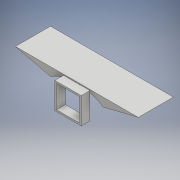
# Autodesk Inventor part: RescueKitThrow_slope
Saved by Autodesk Inventor 2018.3 (Build 223284000, 284)
## iProperties
Created: 2019-02-15
Part Number: RescueKitThrow_slope
Material: 一般
Document SubType Name: Modeling
Designer: TOMOKI
Density: 1 g/cm^3
Appearance: 既定
Author: TOMOKI
Autodesk Inventor part; units mm, degrees
ref_plane "YZ Plane" through (0, 0, 0) normal (1, 0, 0) x (0, 1, 0)
ref_plane "XZ Plane" through (0, 0, 0) normal (0, 1, 0) x (-1, 0, 0)
ref_plane "XY Plane" through (0, 0, 0) normal (0, 0, 1) x (1, 0, 0)
sketch "スケッチ1" plane through (0, 0, 0) normal (0, 1, 0) x (-1, 0, 0)
  line L0 (55, 0) -> (85, 0)
  line L1 (57, -2) -> (83, -2)
  line L2 (83, -2) -> (83, -28)
  line L3 (83, -28) -> (57, -28)
  line L4 (57, -28) -> (57, -2)
  line L5 (85, -30) -> (55, -30)
  line L6 (55, -30) -> (55, 0)
  line L7 (85, 0) -> (85, -30)
  point P0 (0, 0)
  dimension "d15" = 30
  constraints: 16 end point
  measures "d15" distance of L0.end L0.start
extrude "押し出し1" add sketch "スケッチ1" along normal blind 10
sketch "スケッチ3" plane through (0, 10, 0) normal (0, 1, 0) x (1, 0, 0)
  line L0 (0, 0) -> (-140, 0)
  line L1 (0, 0) -> (0, -8.775)
  line L2 (-140, 8.775) -> (-140, 38.775)
  line L3 (-140, 38.775) -> (0, 38.775)
  line L4 (0, 38.775) -> (0, 0)
  line L5 (-140, 0) -> (-140, 38.775)
  line L6 (0, 0) -> (0, 8.775)
  line L7 (0, 8.775) -> (-40.1965, 8.775)
  line L8 (0, 8.775) -> (-40.1965, 8.775)
  line L9 (-99.8035, 8.775) -> (-140, 8.775)
  line L10 (-99.8035, 8.775) -> (-140, 8.775)
  arc A0 (-99.8035, 8.775) -> (-40.1965, 8.775) centre (-70, 55) ccw
  point P0 (-140, -38.775)
  point P1 (-40.1965, -8.775)
  constraints: 22 end point, 3 symmetric about line, 2 point on circle, 1 centre point, 1 point on line
extrude "押し出し2" add sketch "スケッチ3" along normal blind 40 contours L0 A0 L7 L4 | L0 L5 L9 A0
sketch "スケッチ4" plane through (0, 10, 0) normal (0, 0, 1) x (1, 0, 0)
  line L0 (0, 40) -> (-140, 40)
  line L1 (-140, 40) -> (-140, 0)
  line L2 (-140, 0) -> (0, 0)
  line L3 (0, 0) -> (0, 40)
  point P0 (0, -10)
  constraints: 8 end point, 2 parallel, 1 horizontal, 1 perpendicular
extrude "押し出し3" add sketch "スケッチ4" along normal blind 1
sketch "スケッチ5" plane through (0, 50, 0) normal (0, 1, 0) x (1, 0, 0)
  line L0 (0, -1) -> (0, 8.775) projected
  line L1 (-140, 8.775) -> (-140, -1) projected
  line L2 (-99.8035, 8.775) -> (-140, 8.775) projected
  line L3 (-140, 8.775) -> (-140, -1) projected
  line L4 (0, -1) -> (-140, -1) projected
  line L5 (0, 8.775) -> (0, -1) projected
  line L6 (0, 8.775) -> (-40.1965, 8.775) projected
  arc A0 (-99.8035, 8.775) -> (-40.1965, 8.775) centre (-70, 55) ccw projected
  line L7 (-140, -1) -> (0, -1) projected
  line L8 (-40.1965, 8.775) -> (0, -1)
  arc A1 (-99.8035, 8.775) -> (-40.1965, 8.775) centre (-70, 55) ccw projected
  line L9 (-99.8035, 8.775) -> (-140, -1)
  constraints: 4 end point
extrude "押し出し4" cut sketch "スケッチ5" against normal blind 40 contours L8 L6 L0 | L1 L2 L9
sketch "スケッチ6" plane through (0, 10, 0) normal (0, 1, 0) x (1, 0, 0)
  line L0 (0, -8.775) -> (-40.1965, -8.775) projected
  line L1 (-57, 28) -> (-57, 2) projected
  line L2 (-40.1965, -8.775) -> (-57, -28)
  line L3 (-83, 2) -> (-83, 28) projected
  line L4 (-99.8035, -8.775) -> (-140, 1) projected
  line L5 (-83, -28) -> (-99.8035, -8.775)
  line L6 (-40.1965, -8.775) -> (0, -8.775)
  line L7 (0, -38.775) -> (0, -8.775) projected
  line L8 (-140, -8.775) -> (-140, -38.775) projected
  line L9 (0, -38.775) -> (-140, -38.775)
  line L10 (-140, -38.775) -> (-140, -8.775)
  line L11 (-140, -8.775) -> (-99.8035, -8.775)
  line L12 (0, -38.775) -> (0, -8.775)
  line L13 (-140, -38.775) -> (0, -38.775) projected
  line L14 (-57, -28) -> (-83, -28)
  line L15 (-83, -28) -> (-83, -38.775)
  line L16 (-83, -38.775) -> (-57, -38.775)
  line L17 (-57, -38.775) -> (-57, -28)
  line L18 (0, -38.775) -> (-57, -38.775)
  line L19 (-83, -38.775) -> (-140, -38.775)
  line L20 (-83, -38.775) -> (-140, -38.775)
  line L21 (-83, -28) -> (-83, -38.775)
  line L22 (-40.1965, -8.775) -> (-57, -38.775)
  line L23 (-83, -38.775) -> (-99.8035, -8.775)
  point P0 (0, 0)
  point P1 (-57, -2)
  point P2 (-83, -2)
  constraints: 34 end point, 6 collinear, 3 perpendicular, 2 horizontal, 2 parallel, 1 point on line
extrude "押し出し5" cut sketch "スケッチ6" against normal blind 40 contours L7 L9 L22 L0 | L9 L8 L11 L23
